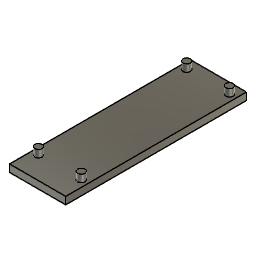
Pressure plate (Autodesk Fusion 360 design; units mm, degrees)
Autodesk Fusion 360 part; units mm, degrees
sketch "Sketch1" plane through (0, 0, 0) normal (0, 0, 1) x (1, 0, 0)
  line L0 (0, 0) -> (23, 0)
  line L1 (23, 0) -> (23, 74)
  line L2 (23, 74) -> (0, 74)
  line L3 (0, 74) -> (0, 0)
  dimension "d1" = 23
  dimension "d2" = 74
  constraint horizontal L0
  constraint vertical L1
  constraint horizontal L2
  constraint vertical L3
  constraint coincident L0.start L3.end
  measures "d1" distance of L0.start L0.end
  measures "d2" distance of L0.start L2.end
extrude "Extrude1" add sketch "Sketch1" along normal blind 3
sketch "Sketch2" plane through (0, 0, 3) normal (0, 0, 1) x (-1, 0, 0)
  line L0 (0, -74) -> (0, 0)
  line L1 (0, 0) -> (-23, 0)
  line L2 (-23, 0) -> (-23, -74)
  line L3 (-23, -74) -> (0, -74)
  circle A0 centre (-2.732, -9.1) radius 1.5
  circle A1 centre (-20.2682, -9.1) radius 1.5
  circle A2 centre (-2.732, -69.81) radius 1.5
  circle A3 centre (-20.2675, -69.81) radius 1.5
  dimension "d5" = 3
  dimension "d6" = 3
  dimension "d7" = 3
  dimension "d8" = 3
  measures "d5" diameter of A0
  measures "d6" diameter of A1
  measures "d7" diameter of A2
  measures "d8" diameter of A3
extrude "Extrude2" add sketch "Sketch2" along normal blind 3 contours A0 | A1 | A2 | A3
